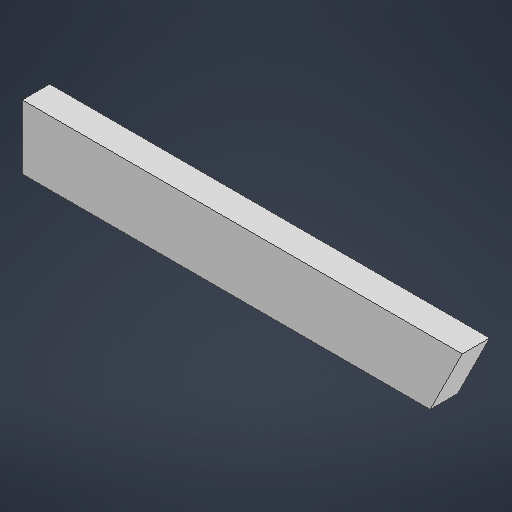
# Autodesk Inventor part: S_2x4x24
Saved by Autodesk Inventor 2026 (Build 300175000, 175)
## iProperties
Created: 2025-09-02
Part Number: S_2x4x24
Material: Generic
Document SubType Name: Modeling
Designer: trott
Density: 1 g/cm^3
Appearance: Default
Author: trott
Autodesk Inventor part; units mm, degrees
ref_plane "YZ Plane" through (0, 0, 0) normal (1, 0, 0) x (0, 1, 0)
ref_plane "XZ Plane" through (0, 0, 0) normal (0, 1, 0) x (-1, 0, 0)
ref_plane "XY Plane" through (0, 0, 0) normal (0, 0, 1) x (1, 0, 0)
sketch "Sketch1" plane through (0, 0, 0) normal (0, 0, 1) x (1, 0, 0)
  line L0 (0, 0) -> (0, -1219.2)
  line L1 (0, 0) -> (609.6, 0)
  line L2 (609.6, 0) -> (0, -1219.2)
  line L3 (0, 0) -> (0, -88.9)
  line L4 (0, -88.9) -> (565.15, -88.9)
  dimension "d8" = 1219.2
  dimension "d9" = 609.6
  dimension "d10" = 88.9
  constraints: 10 end point, 2 point on line, 1 horizontal, 1 perpendicular, 1 vertical
  measures "d8" distance of L0.start L0.end
  measures "d9" distance of L0.start L1.end
  measures "d10" distance of L0.start L3.end
extrude "Extrusion1" add sketch "Sketch1" along normal blind 38.1 contours L1 L2 L4 L0
body "Solid1"
